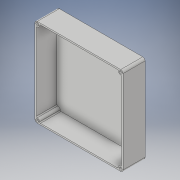
# Autodesk Inventor part: electronics_box_small
Saved by Autodesk Inventor 2019.4 (Build 234330000, 330)
## iProperties
Created: 2020-10-01
Part Number: electronics_box_small
Material: Generic
Document SubType Name: Modeling
Designer: deanv
Density: 1 g/cm^3
Appearance: Default
Author: deanv
Autodesk Inventor part; units mm, degrees
ref_plane "YZ Plane" through (0, 0, 0) normal (1, 0, 0) x (0, 1, 0)
ref_plane "XZ Plane" through (0, 0, 0) normal (0, 1, 0) x (-1, 0, 0)
ref_plane "XY Plane" through (0, 0, 0) normal (0, 0, 1) x (1, 0, 0)
sketch "Sketch1" plane through (0, 0, 0) normal (0, 0, 1) x (1, 0, 0)
  line L0 (-75, -75) -> (75, -75)
  line L1 (75, -75) -> (75, 75)
  line L2 (75, 75) -> (-75, 75)
  line L3 (-75, 75) -> (-75, -75)
  line L4 (-75, -75) -> (75, 75) construction
  line L5 (75, -75) -> (-75, 75) construction
  line L6 (72.5, -72.5) -> (-72.5, -72.5)
  line L7 (-72.5, -72.5) -> (-72.5, 72.5)
  line L8 (-72.5, 72.5) -> (72.5, 72.5)
  line L9 (72.5, 72.5) -> (72.5, -72.5)
  line L10 (72.5, -72.5) -> (-72.5, 72.5) construction
  line L11 (-72.5, -72.5) -> (72.5, 72.5) construction
  line L12 (-75, 75) -> (-71, 75) construction
  line L13 (-71, 75) -> (-71, 71) construction
  line L14 (-71, 71) -> (-75, 71) construction
  line L15 (-75, 71) -> (-75, 75) construction
  circle A0 centre (-71, 71) radius 2.5
  line L16 (-71, -71) -> (-71, -75) construction
  line L17 (-75, -71) -> (-71, -71) construction
  circle A1 centre (-71, -71) radius 2.5
  line L18 (72.5, 72.5) -> (-72.5, -72.5) construction
  line L19 (75, 75) -> (-75, -75) construction
  line L20 (71, -71) -> (75, -71) construction
  line L21 (71, -75) -> (71, -71) construction
  circle A2 centre (71, -71) radius 2.5
  line L22 (-72.5, 72.5) -> (72.5, -72.5) construction
  line L23 (-75, 75) -> (75, -75) construction
  line L24 (71, 71) -> (71, 75) construction
  line L25 (75, 71) -> (71, 71) construction
  circle A3 centre (71, 71) radius 2.5
  line L26 (-72.5, -72.5) -> (72.5, 72.5) construction
  line L27 (-75, -75) -> (75, 75) construction
  line L28 (-73.5, 73.5) -> (-68.5, 73.5)
  line L29 (-68.5, 73.5) -> (-68.5, 68.5)
  line L30 (-68.5, 68.5) -> (-73.5, 68.5)
  line L31 (-73.5, 68.5) -> (-73.5, 73.5)
  line L32 (-73.5, 73.5) -> (-68.5, 68.5) construction
  line L33 (-68.5, 73.5) -> (-73.5, 68.5) construction
  line L34 (-72.5, -72.5) -> (72.5, 72.5) construction
  line L35 (72.5, 72.5) -> (-72.5, -72.5) construction
  line L36 (-75, -75) -> (75, 75) construction
  line L37 (75, 75) -> (-75, -75) construction
  line L38 (-73.5, -68.5) -> (-68.5, -68.5)
  line L39 (-73.5, -73.5) -> (-68.5, -68.5) construction
  line L40 (-68.5, -68.5) -> (-68.5, -73.5)
  line L41 (-68.5, -73.5) -> (-73.5, -73.5)
  line L42 (-73.5, -73.5) -> (-73.5, -68.5)
  line L43 (72.5, -72.5) -> (-72.5, 72.5) construction
  line L44 (-72.5, 72.5) -> (72.5, -72.5) construction
  line L45 (75, -75) -> (-75, 75) construction
  line L46 (-75, 75) -> (75, -75) construction
  line L47 (68.5, -73.5) -> (68.5, -68.5)
  line L48 (73.5, -73.5) -> (68.5, -68.5) construction
  line L49 (68.5, -68.5) -> (73.5, -68.5)
  line L50 (73.5, -68.5) -> (73.5, -73.5)
  line L51 (73.5, -73.5) -> (68.5, -73.5)
  line L52 (72.5, 72.5) -> (-72.5, -72.5) construction
  line L53 (-72.5, -72.5) -> (72.5, 72.5) construction
  line L54 (75, 75) -> (-75, -75) construction
  line L55 (-75, -75) -> (75, 75) construction
  line L56 (73.5, 68.5) -> (68.5, 68.5)
  line L57 (73.5, 73.5) -> (68.5, 68.5) construction
  line L58 (68.5, 68.5) -> (68.5, 73.5)
  line L59 (68.5, 73.5) -> (73.5, 73.5)
  line L60 (73.5, 73.5) -> (73.5, 68.5)
  line L61 (-72.5, 68.5) -> (-72.5, 67)
  line L62 (-72.5, 67) -> (-67, 67)
  line L63 (-67, 67) -> (-67, 72.5)
  line L64 (-67, 72.5) -> (-68.5, 72.5)
  line L65 (-68.5, 72.5) -> (-68.5, 68.5)
  line L66 (-68.5, 68.5) -> (-72.5, 68.5)
  line L67 (-67, -67) -> (-72.5, -67)
  line L68 (-67, -72.5) -> (-67, -67)
  line L69 (72.5, 72.5) -> (-72.5, -72.5) construction
  line L70 (72.5, 72.5) -> (-72.5, -72.5) construction
  line L71 (-72.5, -72.5) -> (72.5, 72.5) construction
  line L72 (-72.5, -72.5) -> (72.5, 72.5) construction
  line L73 (-75, -75) -> (75, 75) construction
  line L74 (-75, -75) -> (75, 75) construction
  line L75 (75, 75) -> (-75, -75) construction
  line L76 (75, 75) -> (-75, -75) construction
  line L77 (67, -67) -> (67, -72.5)
  line L78 (72.5, -67) -> (67, -67)
  line L79 (-72.5, 72.5) -> (72.5, -72.5) construction
  line L80 (-72.5, 72.5) -> (72.5, -72.5) construction
  line L81 (72.5, -72.5) -> (-72.5, 72.5) construction
  line L82 (72.5, -72.5) -> (-72.5, 72.5) construction
  line L83 (75, -75) -> (-75, 75) construction
  line L84 (75, -75) -> (-75, 75) construction
  line L85 (-75, 75) -> (75, -75) construction
  line L86 (-75, 75) -> (75, -75) construction
  line L87 (67, 67) -> (72.5, 67)
  line L88 (67, 72.5) -> (67, 67)
  line L89 (-72.5, -72.5) -> (72.5, 72.5) construction
  line L90 (-72.5, -72.5) -> (72.5, 72.5) construction
  line L91 (72.5, 72.5) -> (-72.5, -72.5) construction
  line L92 (72.5, 72.5) -> (-72.5, -72.5) construction
  line L93 (75, 75) -> (-75, -75) construction
  line L94 (75, 75) -> (-75, -75) construction
  line L95 (-75, -75) -> (75, 75) construction
  line L96 (-75, -75) -> (75, 75) construction
  line L97 (-72.5, -67) -> (-72.5, -68.5)
  line L98 (-72.5, -68.5) -> (-68.5, -68.5)
  line L99 (-68.5, -68.5) -> (-68.5, -72.5)
  line L100 (-68.5, -72.5) -> (-67, -72.5)
  line L101 (-67, -72.5) -> (-67, -67)
  line L102 (-67, -67) -> (-72.5, -67)
  line L103 (68.5, -72.5) -> (67, -72.5)
  line L104 (67, -72.5) -> (67, -67)
  line L105 (67, -67) -> (72.5, -67)
  line L106 (72.5, -67) -> (72.5, -68.5)
  line L107 (72.5, -68.5) -> (68.5, -68.5)
  line L108 (68.5, -68.5) -> (68.5, -72.5)
  line L109 (67, 72.5) -> (68.5, 72.5)
  line L110 (68.5, 72.5) -> (68.5, 68.5)
  line L111 (68.5, 68.5) -> (72.5, 68.5)
  line L112 (72.5, 68.5) -> (72.5, 67)
  line L113 (72.5, 67) -> (67, 67)
  line L114 (67, 67) -> (67, 72.5)
  point P0 (0, 0)
  point P1 (0, 0)
  point P2 (0, 0)
  point P3 (0, 0)
  point P4 (0, 0)
  point P5 (0, 0)
  point P6 (0, 0)
  point P7 (0, 0)
  point P8 (0, 0)
  point P9 (0, 0)
  point P10 (0, 0)
  point P11 (0, 0)
  point P12 (0, 0)
  point P13 (0, 0)
  point P14 (0, 0)
  point P15 (0, 0)
  point P16 (0, 0)
  point P17 (0, 0)
  point P18 (-68.5, 68.5)
  point P19 (0, 0)
  point P20 (0, 0)
  point P21 (0, 0)
  point P22 (0, 0)
  point P23 (-68.5, -68.5)
  dimension "d0" = 150
  dimension "d1" = 150
  dimension "d2" = 145
  dimension "d3" = 145
  dimension "d8" = 4
  dimension "d9" = 4
  dimension "d10" = 5
  dimension "d13" = 360
  dimension "d17" = 360
  dimension "d25" = 1.5
  dimension "d28" = 360
  constraints: 230 end point, 51 midpoint, 36 point on line, 11 coincident, 9 perpendicular, 8 parallel, 7 collinear, 4 centre point, 4 horizontal, 1 tangent, 295 other
  measures "d0" distance of L2.end L1.end
  measures "d1" distance of L1.end L0.end
  measures "d2" distance of L7.end L8.end
  measures "d3" distance of L6.end L7.end
  measures "d8" distance of L13.end L14.end
  measures "d9" distance of L12.end L13.end
  measures "d10" diameter of A0
  measures "d25" distance of L61.start L61.end
extrude "Extrusion1" add sketch "Sketch1" along normal blind 2.5 contours L47 A2 L6 | L6 L77 L78 L9 L49 L47 | L6 L68 L67 L7 L62 L63 L8 L88 L87 L9 L78 L77 | A2 L9 L6 | L47 L49 A2 | L6 L40 L38 L7 L67 L68 | L49 L9 A2 | L6 A1 L40 | L6 L7 A1 | A1 L38 L40 | L87 L88 L8 L58 L56 L9 | A1 L7 L38 | L7 L30 L29 L8 L63 L62 | L56 A3 L9 | L7 A0 L30 | A3 L8 L9 | L56 L58 A3 | L7 L8 A0 | A0 L29 L30 | L58 L8 A3 | A0 L8 L29 picked at (70.3289, -70.3289) picked at (-70.3289, -70.3289) picked at (70.3289, 70.3289) picked at (-70.3289, 70.3289)
extrude "Extrusion2" add sketch "Sketch1" along normal blind 37.5 contours L3 L2 L1 L0 | L6 A2 L51 L47 | L6 L9 A2 | A2 L50 L51 | L40 L41 A1 L6 | L9 L49 L50 A2 | A1 L7 L6 | L41 L42 A1 | L7 A1 L42 L38 | L9 A3 L60 L56 | L30 L31 A0 L7 | L9 L8 A3 | A0 L8 L7 | A3 L59 L60 | L58 L59 A3 L8 | L31 L28 A0 | L8 A0 L28 L29 picked at (72.6398, -70.2994) picked at (-72.6398, -70.2994) picked at (72.6398, 70.2994) picked at (-72.6398, 70.2994)
extrude "Extrusion3" add sketch "Sketch1" along normal blind 37.5 contours L47 A2 L6 | L6 A2 L51 L47 | A2 L9 L6 | L6 L9 A2 | L47 L49 A2 | A2 L50 L51 | L49 L9 A2 | L40 L41 A1 L6 | L6 A1 L40 | L9 L49 L50 A2 | A1 L7 L6 | L6 L7 A1 | A1 L38 L40 | L41 L42 A1 | A1 L7 L38 | L7 A1 L42 L38 | L56 A3 L9 | L9 A3 L60 L56 | L30 L31 A0 L7 | L7 A0 L30 | A3 L8 L9 | L9 L8 A3 | L56 L58 A3 | A0 L8 L7 | L7 L8 A0 | A0 L29 L30 | A3 L59 L60 | L58 L8 A3 | L58 L59 A3 L8 | L31 L28 A0 | A0 L8 L29 | L8 A0 L28 L29
extrude "Extrusion4" cut sketch "Sketch1" along normal blind 37.5 contours A2 L9 L6 | L6 L9 A2 | A1 L7 L6 | L6 L7 A1 | A3 L8 L9 | L9 L8 A3 | A0 L8 L7 | L7 L8 A0
extrude "Extrusion5" add sketch "Sketch1" along normal blind 35.5 contours A2 L9 L6 | L6 L9 A2 | A1 L7 L6 | L6 L7 A1 | A3 L8 L9 | L9 L8 A3 | A0 L8 L7 | L7 L8 A0
extrude "Extrusion6" add sketch "Sketch1" along normal blind 37.5 contours L47 A2 L6 | L6 A2 L51 L47 | L6 L77 L78 L9 L49 L47 | L6 L68 L67 L7 L62 L63 L8 L88 L87 L9 L78 L77 | A2 L9 L6 | L6 L9 A2 | L47 L49 A2 | L6 L40 L38 L7 L67 L68 | A2 L50 L51 | L49 L9 A2 | L40 L41 A1 L6 | L6 A1 L40 | L9 L49 L50 A2 | A1 L7 L6 | L6 L7 A1 | A1 L38 L40 | L87 L88 L8 L58 L56 L9 | L41 L42 A1 | A1 L7 L38 | L7 A1 L42 L38 | L7 L30 L29 L8 L63 L62 | L56 A3 L9 | L9 A3 L60 L56 | L30 L31 A0 L7 | L7 A0 L30 | A3 L8 L9 | L9 L8 A3 | L56 L58 A3 | A0 L8 L7 | L7 L8 A0 | A0 L29 L30 | A3 L59 L60 | L58 L8 A3 | L58 L59 A3 L8 | L31 L28 A0 | A0 L8 L29 | L8 A0 L28 L29
extrude "Extrusion7" cut sketch "Sketch1" along normal blind 37.5 contours L6 L68 L67 L7 L62 L63 L8 L88 L87 L9 L78 L77 | A2 L9 L6 | L6 L9 A2 | A1 L7 L6 | L6 L7 A1 | A3 L8 L9 | L9 L8 A3 | A0 L8 L7 | L7 L8 A0
extrude "Extrusion8" add sketch "Sketch1" along normal blind 2.5 contours L47 A2 L6 | L6 A2 L51 L47 | L6 L77 L78 L9 L49 L47 | L6 L68 L67 L7 L62 L63 L8 L88 L87 L9 L78 L77 | A2 L9 L6 | L6 L9 A2 | L47 L49 A2 | L6 L40 L38 L7 L67 L68 | A2 L50 L51 | L49 L9 A2 | L40 L41 A1 L6 | L6 A1 L40 | L9 L49 L50 A2 | A1 L7 L6 | L6 L7 A1 | A1 L38 L40 | L87 L88 L8 L58 L56 L9 | L41 L42 A1 | A1 L7 L38 | L7 A1 L42 L38 | L7 L30 L29 L8 L63 L62 | L56 A3 L9 | L9 A3 L60 L56 | L30 L31 A0 L7 | L7 A0 L30 | A3 L8 L9 | L9 L8 A3 | L56 L58 A3 | A0 L8 L7 | L7 L8 A0 | A0 L29 L30 | A3 L59 L60 | L58 L8 A3 | L58 L59 A3 L8 | L31 L28 A0 | A0 L8 L29 | L8 A0 L28 L29
extrude "Extrusion9" add sketch "Sketch1" along normal blind 35.5 contours A2 L9 L6 | L6 L9 A2 | A1 L7 L6 | L6 L7 A1 | A3 L8 L9 | L9 L8 A3 | A0 L8 L7 | L7 L8 A0
fillet "Fillet1" radius 4 4 edges at (-75, -75, 18.75) (75, -75, 18.75) (75, 75, 18.75) (-75, 75, 18.75)
fillet "Fillet2" radius 4 4 edges at (-67, 67, 20) (-67, -67, 20) (67, 67, 20) (67, -67, 20)
fillet "Fillet3" radius 1.5 8 edges at (-67, 72.5, 20) (-72.5, 67, 20) (67, 72.5, 20) (72.5, 67, 20) (67, -72.5, 20) (72.5, -67, 20) (-72.5, -67, 20) (-67, -72.5, 20)
body "Solid1"
